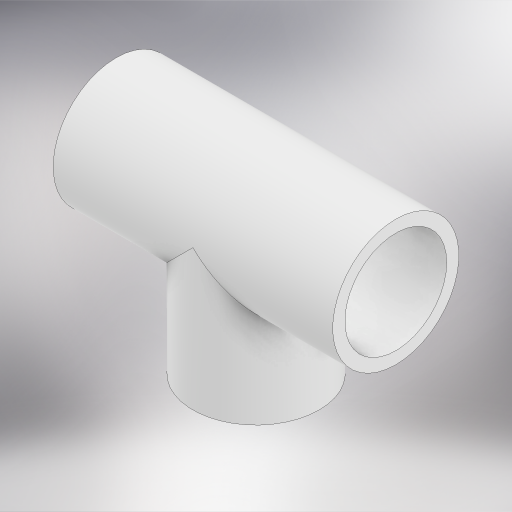
# Autodesk Inventor part: T
Saved by Autodesk Inventor 2023 (Build 270158000, 158)
## iProperties
Created: 2023-02-27
Part Number: T
Material: PVC, no plastificado
Document SubType Name: Modeling
Designer: Braya
Density: 1.29 g/cm^3
Appearance: Suave - Blanco
Mass: 34.8769 g
Surface Area: 178.963 cm^2
Volume: 27.0363 cm^3
Author: Braya
Autodesk Inventor part; units mm, degrees
ref_plane "YZ Plane" through (0, 0, 0) normal (1, 0, 0) x (0, 1, 0)
ref_plane "XZ Plane" through (0, 0, 0) normal (0, 1, 0) x (-1, 0, 0)
ref_plane "XY Plane" through (0, 0, 0) normal (0, 0, 1) x (1, 0, 0)
sketch "Boceto2" plane through (0, 0, 0) normal (0, 1, 0) x (-1, 0, 0)
  circle A0 centre (0, 0) radius 16.5
  dimension "d0" = 33
  constraints: 1 centre point, 1 coincident
  measures "d0" diameter of A0
extrude "Extrusión1" add sketch "Boceto2" along normal blind 36.8
sketch "Boceto3" plane through (0, 0, 0) normal (1, 0, 0) x (0, 1, 0)
  line L0 (0, 0) -> (36.8, 0)
  line L1 (36.8, -16.5) -> (36.8, 16.5) projected
  circle A0 centre (36.8, 0) radius 16.5
  constraints: 2 end point, 1 coincident, 1 midpoint, 1 vertical alignment, 2 other
extrude "Extrusión2" add sketch "Boceto3" along normal mid plane 73.14
sketch "Boceto4" plane through (36.57, 36.8, 0) normal (1, 0, 0) x (0, 0, -1)
  circle A0 centre (0, 0) radius 13.325
  point P0 (0, -36.8)
  dimension "d5" = 26.65
  constraints: 1 centre point
  measures "d5" diameter of A0
extrude "Extrusión3" cut sketch "Boceto4" against normal blind 73.14
sketch "Boceto5" plane through (0, 0, 0) normal (0, -1, 0) x (1, 0, 0)
  circle A0 centre (0, 0) radius 13.325
  dimension "d8" = 26.65
  constraints: 1 centre point, 1 coincident
  measures "d8" diameter of A0
extrude "Extrusión4" cut sketch "Boceto5" against normal up to surface
